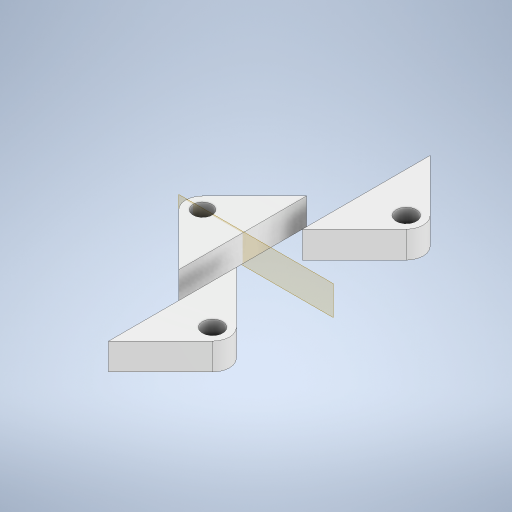
# Autodesk Inventor part: Soporte Rieles - Antenas
Saved by Autodesk Inventor 2023 (Build 270158000, 158)
## iProperties
Created: 2023-11-07
Part Number: Soporte Rieles - Antenas
Material: ABS Plastic
Document SubType Name: Modeling
Designer: juanp
Density: 1.06 g/cm^3
Appearance: Smooth - White
Author: juanp
Autodesk Inventor part; units mm, degrees
ref_plane "YZ Plane" through (0, 0, 0) normal (1, 0, 0) x (0, 1, 0)
ref_plane "XZ Plane" through (0, 0, 0) normal (0, 1, 0) x (-1, 0, 0)
sketch "Sketch1" plane through (0, 0, 0) normal (0, 1, 0) x (-1, 0, 0)
  line L0 (10, 145) -> (-10, 145) construction
  line L1 (-10, 145) -> (-10, -145)
  line L2 (-10, -145) -> (10, -145) construction
  line L3 (10, -145) -> (10, 145)
  line L4 (10, 145) -> (-10, -145) construction
  line L5 (-10, 145) -> (10, -145) construction
  line L6 (10, 0) -> (10, 145)
  line L7 (10, 72.5) -> (40, 72.5) construction
  line L8 (-10, 0) -> (-10, -145) construction
  line L9 (-10, -72.5) -> (-40, -72.5) construction
  line L10 (40, 72.5) -> (-40, 72.5) construction
  line L11 (-40, 72.5) -> (-40, -72.5) construction
  line L12 (-40, -72.5) -> (40, -72.5) construction
  line L13 (40, -72.5) -> (40, 72.5) construction
  circle A0 centre (40, 72.5) radius 7.6 construction
  circle A1 centre (-40, 72.5) radius 7.6
  circle A2 centre (-40, -72.5) radius 7.6
  circle A3 centre (40, -72.5) radius 7.6 construction
  circle A4 centre (40, 0) radius 7.1
  circle A5 centre (-40, 72.5) radius 12.6
  circle A6 centre (-40, -72.5) radius 12.6
  circle A7 centre (40, 0) radius 12.6
  line L14 (48.9095, 8.9095) -> (10, 47.8191)
  line L15 (48.9095, -8.9095) -> (10, -47.8191)
  line L16 (-48.9095, 81.4095) -> (-10, 120.3191)
  line L17 (-48.9095, 63.5905) -> (-10, 24.6809)
  line L18 (-48.9095, -63.5905) -> (-10, -24.6809)
  line L19 (-48.9095, -81.4095) -> (-10, -120.3191)
  point P0 (0, 0)
  point P1 (-10, -120.3191)
  point P2 (10, 47.8191)
  dimension "d0" = 20
  dimension "d1" = 290
  dimension "d2" = 80
  dimension "d3" = 15.2
  dimension "d4" = 14.2
  dimension "d5" = 5
  dimension "d6" = 45
  dimension "d7" = 45
  dimension "d8" = 45
  dimension "d9" = 45
  dimension "d10" = 45
  dimension "d11" = 45
  constraints: 40 end point, 8 centre point, 7 coincident, 7 midpoint, 6 point on circle, 6 point on line, 6 tangent, 5 equal radius, 5 parallel, 4 horizontal, 2 perpendicular, 1 collinear, 1 vertical
  measures "d0" distance of L2.end L1.end
  measures "d1" distance of L1.end L0.end
  measures "d2" distance of L9.end L12.end
  measures "d3" diameter of A0
  measures "d4" diameter of A4
  measures "d5" radial gap between concentric circles of A2 A6
  measures "d6" angle of L14 L3
  measures "d7" angle of L15 L3
  measures "d8" angle of L1 L16
  measures "d9" angle of L1 L17
  measures "d10" angle of L1 L18
  measures "d11" angle of L8 L19
extrude "Extrusion1" add sketch "Sketch1" along normal blind 20
body "Solid1"
